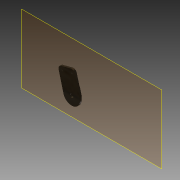
# Autodesk Inventor part: fingerBase01
Saved by Autodesk Inventor 2013 (Build 170138000, 138)
## iProperties
Created: 2014-04-23
Part Number: fingerBase01
Material: Wood (Maple)
Document SubType Name: Modeling
Designer: Nano
Density: 0.57 g/cm^3
Mass: 3.8626 g
Surface Area: 41.3554 cm^2
Volume: 6.7765 cm^3
Author: Nano
Autodesk Inventor part; units mm, degrees
ref_plane "YZ Plane" through (0, 0, 0) normal (1, 0, 0) x (0, 1, 0)
ref_plane "XZ Plane" through (0, 0, 0) normal (0, 1, 0) x (-1, 0, 0)
ref_plane "XY Plane" through (0, 0, 0) normal (0, 0, 1) x (1, 0, 0)
ref_plane "Work Plane1" through (0, 0, 0) normal (0, 0, 1) x (1, 0, 0)
sketch "Sketch1" plane through (0, 0, 0) normal (0, 0, 1) x (1, 0, 0)
  line L0 (-48.9636, -5.919) -> (-45.777, -18.2132)
  arc A0 (-45.777, -18.2132) -> (-22.1173, -12.3142) centre (-33.9472, -15.2637) ccw projected
  line L1 (-22.1173, -12.3142) -> (-25.2457, 0.2285)
  line L2 (-48.9636, -5.919) -> (-25.2457, 0.2285)
  point P0 (0, 0)
  point P1 (-37.0767, -2.9553)
  dimension "d0" = 12.2508
  dimension "d2" = 24.5017
  dimension "d3" = 12.7
  constraints: 6 end point, 1 perpendicular, 1 point on circle
  measures "d0" distance of L0.start point (-37.077, -2.955)
  measures "d2" distance of L0.start L1.end
  measures "d3" distance of A0.centre point (-37.077, -2.955)
extrude "Extrusion1" add sketch "Sketch1" along normal blind 3.175
sketch "Sketch2" plane through (0, 0, 3.175) normal (0, 0, 1) x (1, 0, 0)
  line L0 (-48.9636, -5.919) -> (-45.777, -18.2132) projected
  arc A0 (-45.777, -18.2132) -> (-22.1173, -12.3142) centre (-33.9472, -15.2637) ccw projected
  line L1 (-22.1173, -12.3142) -> (-25.2457, 0.2285) projected
  line L2 (-25.2457, 0.2285) -> (-48.9636, -5.919) projected
  line L3 (-48.9636, -5.919) -> (-45.777, -18.2132) projected
  arc A1 (-45.777, -18.2132) -> (-22.1173, -12.3142) centre (-33.9472, -15.2637) ccw projected
  line L4 (-22.1173, -12.3142) -> (-25.2457, 0.2285) projected
  line L5 (-25.2457, 0.2285) -> (-48.9636, -5.919) projected
  line L6 (-52.8328, -3.6427) -> (-48.8533, -18.9962)
  arc A2 (-48.8533, -18.9962) -> (-19.0376, -11.545) centre (-33.9472, -15.2637) ccw
  line L7 (-19.0376, -11.545) -> (-22.941, 4.1051)
  line L8 (-22.941, 4.1051) -> (-52.8328, -3.6427)
  line L9 (-52.8328, -3.72) -> (-22.941, 4.1051)
  line L10 (-22.941, 4.1051) -> (-29.388, 28.7327)
  line L11 (-29.388, 28.7327) -> (-59.2798, 20.9076)
  line L12 (-59.2798, 20.9076) -> (-52.8328, -3.72)
  point P0 (0, 0)
  constraints: 14 end point, 2 parallel, 2 point on circle, 1 centre point, 1 perpendicular, 3 other
extrude "Extrusion2" add sketch "Sketch2" along normal blind 3.175 contours L2 L1 A0 L0 | L8 L9 L6 | L6 L9 L12 L11 L10 L8 | L9 L7 A2 L6
fillet "Fillet1" radius 6.35 2 edges at (-59.2798, 20.9076, 4.7625) (-29.388, 28.7327, 4.7625)
sketch "Sketch3" plane through (0, 0, 6.35) normal (0, 0, 1) x (1, 0, 0)
  circle A0 centre (-33.9229, -15.2576) radius 3.175
  point P0 (0, 0)
  dimension "d9" = 6.35
  constraints: 1 centre point
  measures "d9" diameter of A0
extrude "Extrusion3" cut sketch "Sketch3" against normal blind 3.175
sketch "Sketch4" plane through (0, 0, 6.35) normal (0, 0, 1) x (1, 0, 0)
  circle A0 centre (-51.5287, 16.3728) radius 1.397
  circle A1 centre (-33.9472, 20.9752) radius 1.397
  point P0 (0, 0)
  dimension "d12" = 2.794
  dimension "d13" = 2.794
  constraints: 2 centre point
  measures "d12" diameter of A0
  measures "d13" diameter of A1
extrude "Extrusion4" cut sketch "Sketch4" against normal up to next
equation "\"d0\" = 0.5 * d2"
body "Solid1"
